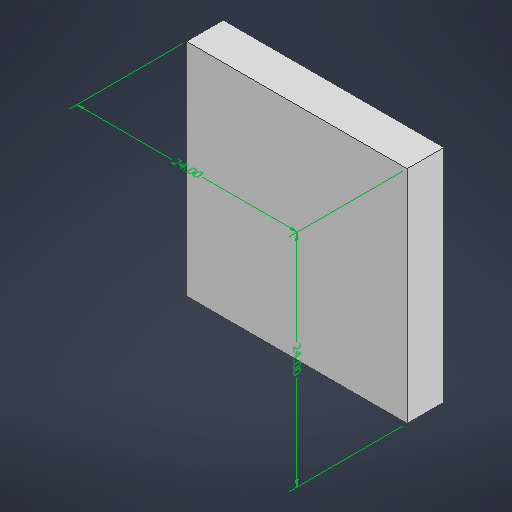
# Autodesk Inventor part: Pieza3
Saved by Autodesk Inventor 2027 (Build 310192000, 192)
## iProperties
Created: 2026-04-02
Part Number: Pieza3
Material: Genérico
Document SubType Name: Modeling
Designer: leand
Density: 1 g/cm^3
Appearance: Valor por defecto
Author: leand
Autodesk Inventor part; units mm, degrees
ref_plane "YZ Plane" through (0, 0, 0) normal (1, 0, 0) x (0, 1, 0)
ref_plane "XZ Plane" through (0, 0, 0) normal (0, 1, 0) x (-1, 0, 0)
ref_plane "XY Plane" through (0, 0, 0) normal (0, 0, 1) x (1, 0, 0)
sketch "Boceto1" plane through (0, 0, 0) normal (0, 0, 1) x (1, 0, 0)
  line L0 (8.3171, 16.6563) -> (32.3171, 16.6563)
  line L1 (32.3171, 16.6563) -> (32.3171, -7.3437)
  line L2 (32.3171, -7.3437) -> (8.3171, -7.3437)
  line L3 (8.3171, -7.3437) -> (8.3171, 16.6563)
  point P0 (0, 0)
  dimension "d0" = 24
  dimension "d1" = 24
  constraints: 8 end point, 2 parallel, 1 horizontal, 1 perpendicular
  measures "d0" distance of L1.end L2.end
  measures "d1" distance of L0.end L1.end
extrude "Extrusión1" add sketch "Boceto1" along normal blind 4
